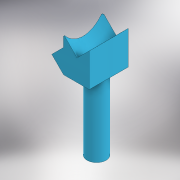
# Autodesk Inventor part: Feed_pin
Saved by Autodesk Inventor 2020 (Build 240168000, 168)
## iProperties
Created: 2020-06-18
Part Number: Feed_pin
Material: Generic
Document SubType Name: Modeling
Designer: pc-konvi
Density: 1 g/cm^3
Appearance: Turquoise
Author: pc-konvi
Autodesk Inventor part; units mm, degrees
ref_plane "YZ Plane" through (0, 0, 0) normal (1, 0, 0) x (0, 1, 0)
ref_plane "XZ Plane" through (0, 0, 0) normal (0, 1, 0) x (-1, 0, 0)
ref_plane "XY Plane" through (0, 0, 0) normal (0, 0, 1) x (1, 0, 0)
sketch "Sketch1" plane through (0, 0, 0) normal (0, 0, 1) x (1, 0, 0)
  line L0 (10.9091, 15) -> (-12.0909, 15)
  line L1 (-12.0909, 15) -> (-12.0909, -15)
  line L2 (-12.0909, -15) -> (10.9091, -15)
  line L3 (10.9091, -15) -> (10.9091, 15)
  line L4 (-12.0909, -15) -> (-22.6975, -4.3934)
  line L5 (-12.0909, -15) -> (2.9091, -15) construction
  line L6 (-22.6975, -4.3934) -> (-12.0909, 6.2132)
  line L7 (-12.0909, 6.2132) -> (2.0731, -7.9508) construction
  line L8 (10.9091, 15.0492) -> (-9.4479, -5.3079) construction
  line L9 (-8.4113, 37.889) -> (15.6041, 13.8735) construction
  line L10 (-5.0089, -0.8688) -> (12.6688, 16.8089)
  line L11 (12.6688, 16.8089) -> (-8.4113, 37.889)
  line L12 (-8.4113, 37.889) -> (-26.089, 20.2113)
  line L13 (-26.089, 20.2113) -> (-5.0089, -0.8688)
  point P0 (0, 0)
  point P1 (10.9091, 0)
  dimension "d0" = 30
  dimension "d1" = 23
  dimension "d2" = 15
  dimension "d3" = 135
  dimension "d4" = 15
  dimension "d5" = 25
  constraints: 28 end point, 5 parallel, 5 point on line, 3 perpendicular, 2 horizontal, 2 midpoint, 1 equal length, 1 horizontal alignment
  measures "d0" distance of L2.end L0.start
  measures "d1" distance of L1.end L2.end
  measures "d2" distance of L1.end L4.end
  measures "d3" angle of L5 L4
  measures "d4" distance of L4.end L6.end
  measures "d5" distance between parallel lines of L7 L9
extrude "Extrusion1" add sketch "Sketch1" along normal mid plane 35 contours L3 L2 L1 L13 L10 L0 | L10 L13 L1 L0 | L4 L6 L1
revolve "Revolution1" cut sketch "Sketch1" angle 360 about axis through (12.6688, 16.8089, 0) along (-0.7071, 0.7071, 0) contours L10 L13 L1 L0 | L0 L1 L13 L12 L11 L10
sketch "Sketch2" plane through (-12.0909, -15, 17.5) normal (0, -1, 0) x (1, 0, 0)
  circle A0 centre (12.0909, -17.5) radius 8.5
  dimension "d9" = 17
  constraints: 1 centre point, 1 coincident
  measures "d9" diameter of A0
extrude "Extrusion2" add sketch "Sketch2" along normal blind 65
body "Solid1"
